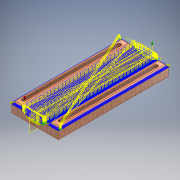
# Autodesk Inventor part: Nameplate Prototype
Saved by Autodesk Inventor 2018 (Build 220112000, 112)
## iProperties
Created: 2017-11-02
Part Number: Nameplate Prototype
Material: Wood (Oak)
Document SubType Name: Modeling
Designer: 223171
Density: 0.76 g/cm^3
Appearance: White Oak - Natural Medium Gloss
Author: 223171
Autodesk Inventor part; units mm, degrees
ref_plane "YZ Plane" through (0, 0, 0) normal (1, 0, 0) x (0, 1, 0)
ref_plane "XZ Plane" through (0, 0, 0) normal (0, 1, 0) x (-1, 0, 0)
ref_plane "XY Plane" through (0, 0, 0) normal (0, 0, 1) x (1, 0, 0)
sketch "Sketch2" plane through (0, 0, 0) normal (0, 0, 1) x (1, 0, 0)
  line L0 (0, 0) -> (85, 0)
  line L1 (85, 0) -> (85, -200)
  line L2 (85, -200) -> (0, -200)
  line L3 (0, -200) -> (0, 0)
  dimension "d0" = 85
  dimension "d1" = 200
  constraints: 8 end point, 2 parallel, 1 horizontal, 1 perpendicular
  measures "d0" distance of L1.end L2.end
  measures "d1" distance of L0.end L1.end
extrude "Extrusion1" add sketch "Sketch2" along normal blind 19
sketch "Sketch3" plane through (10, -200, 0) normal (0, -1, 0) x (1, 0, 0)
  line L0 (75, 19) -> (-10, 19) projected
  line L1 (7.5, 19) -> (57.5, 19) construction
  spline S0 degree 1 poles (7.5, 19) (57.5, 19) knots 1 1 2 2
  spline S1 degree 2 poles (7.5, 19) (33.1045, -4.0017) (57.5, 19) knots 0 0 0 1 1 1
  line L2 (75, 0) -> (-10, 0) projected
  line L3 (0, 0) -> (0, 19) projected
  line L4 (65, 19) -> (65, 0) projected
  point P0 (33.0146, 7.5)
  dimension "d5" = 7.5
  dimension "d6" = 7.5
  dimension "d7" = 7.5
  constraints: 2 point on line, 6 other
  measures "d5" distance from line of L2 point (33.015, 7.5)
  measures "d6" distance from line of L3 L1.start
  measures "d7" distance from line of L4 L1.end
extrude "Extrusion2" cut sketch "Sketch3" against normal through all contours S1 L0
chamfer "Chamfer1" distance 3 angle 45 8 edges at (0, -100, 19) (76.25, -200, 19) (8.75, -200, 19) (67.5, -100, 19) (17.5, -100, 19) (76.25, 0, 19) (8.75, 0, 19) (85, -100, 19)
sketch "Sketch11" plane through (0, 0, 19) normal (0, 0, 1) x (1, 0, 0)
  line L0 (28.5921, -198.4024) -> (28.5921, -3.1228) construction
  line L1 (28.5921, -3.1228) -> (55.2331, -3.1228) construction
  line L2 (55.2331, -3.1228) -> (55.2331, -198.4024) construction
  line L3 (55.2331, -198.4024) -> (28.5921, -198.4024) construction
  line L4 (72.75, -190.2199) -> (79.499, -190.2199)
  line L5 (79.499, -190.2199) -> (79.499, -10)
  line L6 (79.499, -10) -> (72.75, -10)
  line L7 (72.75, -10) -> (72.75, -190.2199)
  point P0 (0, 0)
  dimension "d30" = 6.749
  constraints: 8 end point, 2 parallel, 1 horizontal, 1 perpendicular, 2 other
  measures "d30" distance between parallel lines of L5 L7
extrude "Extrusion5" cut sketch "Sketch11" against normal blind 5
ref_plane "Work Plane1" through (42.5, -190, 0) normal (1, 0, 0) x (0, 0, -1)
mirror "Mirror1" about plane through (42.5, -190, 0) normal (1, 0, 0) of "Extrusion5"
fillet "Fillet3" radius 3 8 edges at (5.501, -10, 16.5) (72.75, -10, 16.5) (79.499, -10, 16.5) (12.25, -10, 16.5) (72.75, -190.2199, 16.5) (5.501, -190.2199, 16.5) (79.499, -190.2199, 16.5) (12.25, -190.2199, 16.5)
body "Solid1"
